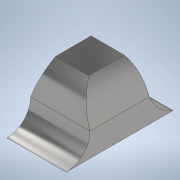
# Autodesk Inventor part: tooth
Saved by Autodesk Inventor 2021 (Build 250183000, 183)
## iProperties
Created: 2021-05-05
Part Number: tooth
Material: Steel, High Strength, Low Alloy
Document SubType Name: Modeling
Density: 7.85 g/cm^3
Appearance: Steel - Polished
Mass: 7.13611 g
Surface Area: 6.44077 cm^2
Volume: 0.909059 cm^3
Autodesk Inventor part; units mm, degrees
ref_plane "YZ Plane" through (0, 0, 0) normal (1, 0, 0) x (0, 1, 0)
ref_plane "XZ Plane" through (0, 0, 0) normal (0, 1, 0) x (-1, 0, 0)
ref_plane "XY Plane" through (0, 0, 0) normal (0, 0, 1) x (1, 0, 0)
sketch "Sketch1" plane through (0, 0, 0) normal (0, 0, 1) x (1, 0, 0)
  line L0 (-5, -2.6054) -> (-5, 1.3946)
  line L1 (-5, -2.6054) -> (0, -2.6054)
  line L2 (0, -2.6054) -> (0, 7.3946)
  line L3 (0, 7.3946) -> (-2.8105, 7.3946)
  line L4 (-2.8105, 7.3946) -> (-5, 1.3946)
  point P0 (0, 0)
  dimension "d0" = 4
  dimension "d1" = 6
  dimension "d2" = 5
  constraints: 10 end point, 2 horizontal, 1 perpendicular, 1 point on line, 1 vertical
  measures "d0" distance of L0.start L0.end
  measures "d1" distance from line of L3 L0.end
  measures "d2" distance of L0.start L1.end
extrude "Extrusion1" add sketch "Sketch1" along normal blind 10
mirror "Mirror1" about plane through (0, 0, 0) normal (1, 0, 0) of "Extrusion1"
sketch "Sketch2" plane through (0, 0, 0) normal (1, 0, 0) x (0, 1, 0)
  line L0 (7.3946, 0) -> (7.3946, 10) projected
  line L1 (7.3946, 10) -> (1.3946, 10) projected
  line L2 (1.3946, 0) -> (1.3946, 10) projected
  arc A0 (7.3946, 8) -> (1.3946, 10) centre (1.3946, 0) ccw
  line L3 (7.3946, 0) -> (1.3946, 0) projected
  arc A1 (1.3946, 0) -> (7.3946, 2) centre (1.3946, 10) ccw
  point P0 (0, 0)
  dimension "d7" = 10
  dimension "d8" = 8
  dimension "d11" = 10
  dimension "d12" = 8
  constraints: 4 point on circle, 2 centre point, 2 point on line
  measures "d7" radius of A0
  measures "d8" vertical distance of point (0, 0) A0.start
  measures "d11" radius of A1
  measures "d12" distance from line of L1 A1.end
extrude "Extrusion3" cut sketch "Sketch2" along normal mid plane 10 contours L3 A1 L0 | A0 L1 L0
sketch "Sketch3" plane through (0, 0, 0) normal (1, 0, 0) x (0, 1, 0)
  line L0 (-2.6054, 0) -> (-2.6054, 10) projected
  line L1 (-2.6054, 10) -> (-2.6054, 14)
  line L2 (1.3946, 0) -> (1.3946, 10) projected
  arc A0 (-2.6054, 14) -> (1.3946, 10) centre (1.3946, 14) ccw
  line L3 (-2.6054, 0) -> (-2.6054, -4)
  line L4 (1.3946, 0) -> (-2.6054, 0) projected
  arc A1 (1.3946, 0) -> (-2.6054, -4) centre (3.9223, -6.5277) ccw
  arc A2 (7.3946, 8) -> (1.3946, 10) centre (1.3946, 0) ccw projected
  point P0 (0, 0)
  dimension "d15" = 4
  dimension "d17" = 7
  dimension "d18" = 4
  constraints: 4 end point, 4 point on circle, 2 centre point, 2 vertical, 1 tangent
  measures "d15" distance of L0.end L1.end
  measures "d17" radius of A1
  measures "d18" distance of L0.start L3.end
extrude "Extrusion4" add sketch "Sketch3" along normal mid plane 10
equation "\"d2\" = rack_tooth_thickness"
equation "\"d3\" = rack_tooth_face_widh"
equation "\"d11\" = d7"
equation "\"d12\" = d8"
equation "\"d17\" = d16"
equation "\"d18\" = d15"
equation "\"rack_tooth_thickness\" = 5"
equation "\"rack_tooth_face_widh\" = 10"
equation "\"rack_tooth_addendum\" = 5"
equation "\"rack_tooth_dedendum\" = 5"
equation "\"hoop_width_large\" = 51"
equation "\"hoop_thickness_large\" = 4"
equation "\"hoop_thickness_small\" = 2"
equation "\"hoop_width_medium\" = 33.7"
equation "\"hoop_thickness_medium\" = 3.2"
equation "\"hoop_width_small\" = 25.4"
equation "\"secure_arm_angle\" = 35deg"
equation "\"secure_arm_radii\" = 9"
equation "\"hoop_bearing_length\" = 5deg"
equation "\"hoop_cable_pulley_diam\" = 22"
equation "\"hoop_cable_diam\" = 5"
equation "\"support_frame_squareBarThickness\" = 5"
equation "\"support_frame_squareBarFillet\" = 2"
equation "\"support_baseClamp_platformThickness\" = 15"
equation "\"support_baseClamp_platformWidthBuffer\" = 0"
equation "\"support_baseClamp_platformLengthBuffer\" = 35"
equation "\"support_frame_endHoleBuffer\" = 45"
equation "\"support_baseClamp_thickness\" = 8"
equation "\"support_baseClamp_sleeveSweepTerminationAngle\" = 55deg"
equation "\"support_baseClamp_sleeveHoleDiameter\" = 12"
equation "\"hoop_angle_z\" = 45deg"
equation "\"hoop_tabs_hole\" = 12"
equation "\"hoop_tabs_thickness\" = 6"
equation "\"wheelchair_deployed_width\" = 635"
equation "\"wheelchair_deployed_height\" = 914"
equation "\"wheelchair_deployed_length\" = 1067"
equation "\"sm_varx_member_tolerance\" = 0"
equation "\"sm_varx_pinPlate_holeDiameter\" = 5"
equation "\"sm_varx_pinPlate_thickness\" = 5"
equation "\"sm_varx_squareBarThickness\" = 2.5"
equation "\"hoop_bushing12_radialInterference\" = 0"
equation "\"hoop_bushing12_od\" = -2 * hoop_thickness_large + hoop_width_large + hoop_bushing12_radialInterference"
equation "\"hoop_bushing23_radialInterference\" = 0"
equation "\"hoop_bushing12_thickness\" = -hoop_width_medium + hoop_bushing12_od - 2 * hoop_bushing12_radialInterference"
equation "\"hoop_bushing23_od\" = -2 * hoop_thickness_medium + hoop_width_medium + hoop_bushing23_radialInterference"
equation "\"hoop_bushing23_thickness\" = -hoop_width_small + hoop_bushing23_od - 2 * hoop_bushing23_radialInterference"
equation "\"wheelchatir_pos_deploy_angle_0\" = 65deg"
equation "\"wheelchatir_pos_store_angle_0\" = 90deg"
equation "\"wheelchatir_pos_deploy_angle_1\" = 20deg"
equation "\"wheelchatir_pos_store_angle_1\" = 20deg"
equation "\"d16\" = 7"
body "Solid1"
